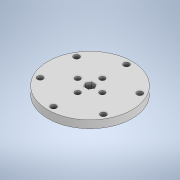
# Autodesk Inventor part: Wheel Mount
Saved by Autodesk Inventor 2020 (Build 240168000, 168)
## iProperties
Created: 2020-01-14
Part Number: Wheel Mount
Material: Generic
Document SubType Name: Modeling
Designer: maple
Density: 1 g/cm^3
Appearance: Default
Author: maple
Autodesk Inventor part; units mm, degrees
ref_plane "YZ Plane" through (0, 0, 0) normal (1, 0, 0) x (0, 1, 0)
sketch "Sketch1" plane through (0, 0, 0) normal (0, 1, 0) x (-1, 0, 0)
  circle A0 centre (0, 0) radius 27.94
  dimension "d0" = 55.88
  constraints: 1 centre point, 1 coincident
  measures "d0" diameter of A0
extrude "Extrusion1" add sketch "Sketch1" along normal blind 7.62
ref_plane "Work Plane5" through (0, 21.082, 0) normal (0, 1, 0) x (1, 0, 0)
sketch "Sketch5" plane through (0, 21.082, 0) normal (0, 1, 0) x (1, 0, 0)
  line L0 (0, 0) -> (0, 2.667)
  line L1 (-3.1168, 0) -> (-1.5584, 2.6992)
  line L2 (-1.5584, 2.6992) -> (1.5584, 2.6992)
  line L3 (1.5584, 2.6992) -> (3.1168, 0)
  line L4 (3.1168, 0) -> (1.5584, -2.6992)
  line L5 (1.5584, -2.6992) -> (-1.5584, -2.6992)
  line L6 (-1.5584, -2.6992) -> (-3.1168, 0)
  dimension "d10" = 2.667
  constraints: 14 end point, 1 coincident, 1 vertical, 13 other
  measures "d10" distance of L0.start L0.end
extrude "Extrusion4" cut sketch "Sketch5" against normal blind 25.4
sketch "Sketch6" plane through (0, 7.62, 0) normal (0, 1, 0) x (1, 0, 0)
  circle A0 centre (0, 0) radius 27.94 projected
  line L0 (0, -27.94) -> (0, -26.162)
  line L1 (0, -26.162) -> (0, -24.257)
  circle A1 centre (0, -24.257) radius 1.905
  dimension "d13" = 1.778
  dimension "d14" = 1.905
  constraints: 4 end point, 2 vertical alignment, 1 coincident, 1 point on line, 1 vertical, 3 other
  measures "d13" distance of L0.start L0.end
  measures "d14" distance of L0.end L1.end
extrude "Extrusion5" cut sketch "Sketch6" against normal blind 25.4 contours A1
ref_plane "Work Plane6" through (0, 21.082, 0) normal (0, 1, 0) x (1, 0, 0)
pattern_circular "Circular Pattern1" count 6 over 360 about axis through (0, 21.082, 0) along (0, 1, 0) of "Extrusion5"
sketch "Sketch8" plane through (0, 0, 0) normal (0, -1, 0) x (1, 0, 0)
  line L0 (3.1168, 0) -> (1.5584, -2.6992) projected
  line L1 (3.1168, 0) -> (6.4188, 0)
  line L2 (6.4188, 0) -> (8.1968, 0)
  circle A0 centre (8.1968, 0) radius 1.778
  point P0 (0, 0)
  dimension "d20" = 3.302
  dimension "d21" = 1.778
  constraints: 4 end point, 2 horizontal, 1 coincident, 1 horizontal alignment, 2 other
  measures "d20" distance of L0.start L1.end
  measures "d21" distance of L1.end L2.end
extrude "Extrusion6" cut sketch "Sketch8" against normal blind 25.4
pattern_circular "Circular Pattern2" count 4 over 360 about axis through (0, 21.082, 0) along (0, 1, 0) of "Extrusion6"
sketch "Sketch10" plane through (0, 7.62, 0) normal (0, 1, 0) x (1, 0, 0)
  circle A0 centre (0, 0) radius 27.94
  constraints: 1 centre point, 1 coincident
extrude "Extrusion8" cut sketch "Sketch10" against normal blind 2.54
body "Solid1"
